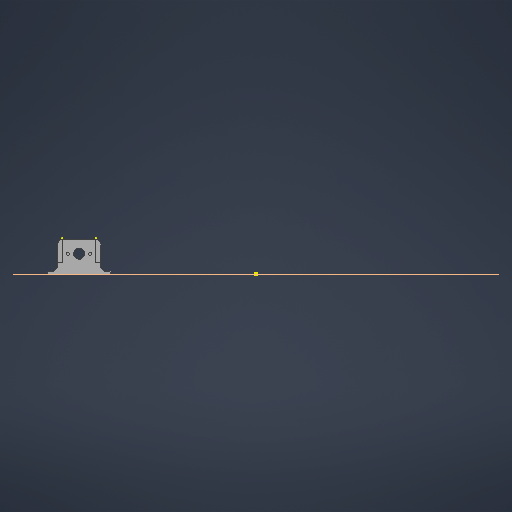
# Autodesk Inventor part: encoder mount
Saved by Autodesk Inventor 2026.1 (Build 301233020, 233B)
## iProperties
Created: 2026-01-21
Part Number: encoder mount
Material: Generic
Document SubType Name: Modeling
Designer: stoof
Density: 1 g/cm^3
Appearance: Default
Author: stoof
Autodesk Inventor part; units mm, degrees
ref_plane "YZ Plane" through (0, 0, 0) normal (1, 0, 0) x (0, 1, 0)
ref_plane "XZ Plane" through (0, 0, 0) normal (0, 1, 0) x (-1, 0, 0)
ref_plane "XY Plane" through (0, 0, 0) normal (0, 0, 1) x (1, 0, 0)
ref_plane "Work Plane1" through (0, 0, 0) normal (0, 0, 1) x (1, 0, 0)
sketch "Sketch1" plane through (0, 0, 0) normal (0, 0, 1) x (1, 0, 0)
  circle A0 centre (24, -114.5) radius 1.15 projected
  circle A1 centre (24, -126.5) radius 1.15 projected
  line L0 (40, -130.5) -> (40, -170.5) projected
  line L1 (30.7, -171.5) -> (21, -171.5)
  line L2 (21, -171.5) -> (21, -109.5)
  line L3 (21, -109.5) -> (30.7, -109.5)
  line L4 (30.7, -109.5) -> (30.7, -171.5)
  line L5 (30.7, -131.5) -> (21, -131.5)
  line L6 (21, -171.5) -> (21, -177.5)
  line L7 (21, -177.5) -> (30.7, -177.5)
  line L8 (30.7, -177.5) -> (30.7, -171.5)
  circle A2 centre (24, -174.5) radius 1.15 projected
  line L9 (21, -123.5) -> (30.7, -123.5)
  point P0 (0, 0)
  point P1 (30.7, -140.5)
  point P2 (21, -140.5)
  dimension "d6" = 9.3
  dimension "d7" = 5
  dimension "d8" = 3
  dimension "d21" = 40
  dimension "d31" = 3
  dimension "d36" = 5
  dimension "d37" = 3
  constraints: 18 end point, 5 perpendicular, 4 point on line, 2 midpoint, 2 parallel, 1 horizontal, 1 vertical
  measures "d6" distance between parallel lines of L0 L4
  measures "d7" distance from line of L3 A0.centre
  measures "d8" distance from line of L2 A0.centre
  measures "d21" distance between parallel lines of L1 L5
  measures "d31" distance from line of L7 A2.centre
  measures "d36" distance from line of L5 A1.centre
  measures "d37" distance from line of A1.centre L9
extrude "Extrusion1" add sketch "Sketch1" along normal blind 2.5 contours L8 L7 L6 L1 | L1 L2 L5 L4 | L5 L2 L9 L4
ref_plane "Work Plane2" through (0, 0, 0) normal (0, 0, 1) x (1, 0, 0)
sketch "Sketch2" plane through (0, 0, 0) normal (0, 0, 1) x (1, 0, 0)
  line L0 (30.7, -171.5) -> (21, -171.5) projected
  line L1 (30.7, -109.5) -> (30.7, -171.5) projected
  line L2 (21, -171.5) -> (21, -109.5) projected
  line L3 (30.7, -131.5) -> (21, -131.5) projected
  line L4 (39.7, -164.8) -> (30.7, -164.8) projected
  line L5 (39.7, -136.2) -> (30.7, -136.2) projected
  line L6 (30.7, -164.8) -> (21, -164.8) construction
  line L7 (30.7, -136.2) -> (21, -136.2) construction
  line L8 (30.7, -132.2) -> (19, -132.2)
  line L9 (30.7, -168.8) -> (19, -168.8)
  point P0 (0, 0)
  point P1 (19, -138)
  point P2 (31, -138)
  point P3 (21, -109.5)
  point P4 (21, -168.8)
  point P5 (30.7, -168.8)
  point P6 (30.7, -132.2)
  point P7 (21, -132.2)
  dimension "d34" = 4
  dimension "d35" = 4
  constraints: 8 end point, 2 horizontal, 2 parallel, 4 other
  measures "d34" distance between parallel lines of L7 L8
  measures "d35" distance between parallel lines of L6 L9
extrude "Extrusion2" add sketch "Sketch2" along normal blind 30 contours L9 L2 L8 L1
sketch "Sketch3" plane through (30.7, -109.5, 2.5) normal (1, 0, 0) x (0, 0, -1)
  arc A0 (-17.7496, -42.5875) -> (-17.7496, -39.4125) centre (-15, -41) ccw projected
  circle A1 centre (-15, -41) radius 4.675
  point P0 (2.5, 109.5)
  dimension "d12" = 1.5
  constraints: 1 centre point, 1 coincident
  measures "d12" radial gap between concentric circles of A0 A1
extrude "Extrusion3" cut sketch "Sketch3" against normal blind 30
sketch "Sketch4" plane through (30.7, -109.5, 2.5) normal (1, 0, 0) x (0, 0, -1)
  circle A0 centre (-15, -41) radius 4.675 projected
  circle A1 centre (-15, -50.525) radius 1.4
  circle A2 centre (-15, -31.475) radius 1.4
  point P0 (2.5, 109.5)
  dimension "d15" = 9.525
  dimension "d16" = 9.525
  dimension "d17" = 2.8
  constraints: 2 centre point, 1 equal radius
  measures "d15" distance of A0.centre A2.centre
  measures "d16" distance of A1.centre A0.centre
  measures "d17" diameter of A1
extrude "Extrusion4" add sketch "Sketch4" along normal blind 3 contours A1 | A2
sketch "Sketch5" plane through (30.7, -109.5, 2.5) normal (1, 0, 0) x (0, 0, -1)
  line L0 (-9.02, -55.3) -> (-28.6471, -55.3) projected
  line L1 (-28.6471, -26.7) -> (-9.02, -26.7) projected
  point P0 (2.5, 109.5)
sketch "Sketch6" plane through (30.7, -109.5, 2.5) normal (1, 0, 0) x (0, 0, -1)
  point P0 (2.5, 109.5)
sketch "Sketch7" plane through (30.7, -109.5, 2.5) normal (1, 0, 0) x (0, 0, -1)
  line L0 (-28.6471, -26.7) -> (-9.02, -26.7) projected
  line L1 (-9.02, -55.3) -> (-28.6471, -55.3) projected
  line L2 (-28.6471, -26.575) -> (-7.5, -26.575)
  line L3 (-7.5, -55.425) -> (-28.6471, -55.425)
  line L4 (-7.5, -26.575) -> (-7.5, -22.7)
  line L5 (-7.5, -59.3) -> (-7.5, -55.425)
  line L6 (0, -59.3) -> (-27.5, -59.3) projected
  line L7 (-27.5, -59.3) -> (-27.5, -22.7) projected
  line L8 (0, -22.7) -> (-27.5, -22.7) projected
  point P0 (2.5, 109.5)
  point P1 (2.5, -62)
  point P2 (-27.5, -26.575)
  point P3 (-27.5, -55.425)
  dimension "d27" = 0.125
  dimension "d28" = 0.125
  constraints: 8 end point, 2 parallel, 2 point on line, 1 perpendicular, 1 vertical
  measures "d27" distance between parallel lines of L0 L2
  measures "d28" distance between parallel lines of L1 L3
extrude "Extrusion5" add sketch "Sketch7" along normal blind 8
sketch "Sketch8" plane through (0, 0, 30) normal (0, 0, 1) x (1, 0, 0)
  line L0 (22.993, -148.2081) -> (27.5704, -148.2081) construction
  line L1 (27.5704, -148.2081) -> (27.5704, -154.4367) construction
  line L2 (27.5704, -154.4367) -> (22.993, -154.4367) construction
  line L3 (22.993, -154.4367) -> (22.993, -148.2081) construction
  line L4 (27.3628, -152.2122) -> (26.6362, -152.2122)
  line L5 (26.6362, -152.2122) -> (26.6362, -154.3081)
  line L6 (26.6362, -154.3081) -> (25.8502, -154.3081)
  line L7 (25.8502, -154.3081) -> (25.8502, -152.2122)
  line L8 (25.8502, -152.2122) -> (23.1561, -152.2122)
  line L9 (23.1561, -152.2122) -> (23.1561, -151.3521)
  line L10 (23.1561, -151.3521) -> (25.8848, -148.2081)
  line L11 (25.8848, -148.2081) -> (26.6362, -148.2081)
  line L12 (26.6362, -148.2081) -> (26.6362, -151.5547)
  line L13 (26.6362, -151.5547) -> (27.3628, -151.5547)
  line L14 (27.3628, -151.5547) -> (27.3628, -152.2122)
  line L15 (25.8502, -151.5547) -> (25.8502, -149.1721)
  line L16 (25.8502, -149.1721) -> (23.7987, -151.5547)
  line L17 (23.7987, -151.5547) -> (25.8502, -151.5547)
  point P0 (0, 0)
  constraints: 2 other
extrude "Extrusion6" cut sketch "Sketch8" against normal blind 0.5
fillet "Fillet3" radius 5 4 edges at (25.85, -168.8, 2.5) (29.85, -168.8, 30) (29.85, -132.2, 30) (25.85, -132.2, 2.5)
body "Solid1"
